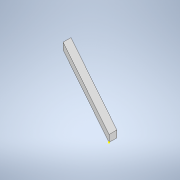
# Autodesk Inventor part: BottomDiagonalSupport
Saved by Autodesk Inventor 2020.1 (Build 241239000, 239)
## iProperties
Created: 2020-02-04
Part Number: BottomDiagonalSupport
Material: Generic
Document SubType Name: Modeling
Designer: super
Density: 1 g/cm^3
Appearance: Default
Author: super
Autodesk Inventor part; units mm, degrees
ref_plane "YZ Plane" through (0, 0, 0) normal (1, 0, 0) x (0, 1, 0)
ref_plane "XZ Plane" through (0, 0, 0) normal (0, 1, 0) x (-1, 0, 0)
ref_plane "XY Plane" through (0, 0, 0) normal (0, 0, 1) x (1, 0, 0)
sketch "Sketch1" plane through (0, 0, 0) normal (0, 1, 0) x (-1, 0, 0)
  point P0 (0, 0)
sketch "Sketch2" plane through (0, 0, 0) normal (0, 1, 0) x (-1, 0, 0)
  line L0 (0, 0) -> (95.3335, -52.8442)
  line L1 (0, 0) -> (109, 0) construction
  line L2 (95.3335, -52.8442) -> (95.3335, -60.1045)
  line L3 (95.3335, -60.1045) -> (0, -7.2603)
  line L4 (0, -7.2603) -> (0, 0)
  dimension "d1" = 29
  constraints: 10 end point, 1 equal length, 1 horizontal, 1 parallel, 1 vertical
  measures "d1" angle of L0 L1
extrude "Extrusion1" add sketch "Sketch2" along normal blind 6.35
body "Solid1"
